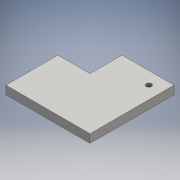
# Autodesk Inventor part: top guide support plate
Saved by Autodesk Inventor 2016 SP1 (Build 200210100, 210)
## iProperties
Created: 2016-05-25
Part Number: top guide support plate
Material: Generic
Document SubType Name: Modeling
Designer: ubik
Density: 1 g/cm^3
Appearance: Default
Author: ubik
Autodesk Inventor part; units mm, degrees
ref_plane "YZ Plane" through (0, 0, 0) normal (1, 0, 0) x (0, 1, 0)
ref_plane "XZ Plane" through (0, 0, 0) normal (0, 1, 0) x (-1, 0, 0)
ref_plane "XY Plane" through (0, 0, 0) normal (0, 0, 1) x (1, 0, 0)
sketch "Sketch1" plane through (0, 0, 0) normal (0, 0, 1) x (1, 0, 0)
  line L0 (-40, 40) -> (40, 40)
  line L1 (40, 40) -> (40, -40)
  line L2 (40, -40) -> (-40, -40)
  line L3 (-40, -40) -> (-40, 40)
  point P0 (0, 0)
  dimension "d0" = 80
  dimension "d1" = 80
  dimension "d4" = 40
  dimension "d5" = 40
  constraints: 8 end point, 2 parallel, 1 horizontal, 1 perpendicular
  measures "d0" distance of L0.start L0.end
  measures "d1" distance of L2.end L0.start
  measures "d4" distance from line of point (0, 0) L3
  measures "d5" distance from line of point (0, 0) L0
extrude "Extrusion1" add sketch "Sketch1" along normal blind 8
sketch "Sketch2" plane through (0, 0, 8) normal (0, 0, 1) x (1, 0, 0)
  circle A0 centre (28, 28) radius 2.5
  line L0 (40, 40) -> (-40, 40) projected
  line L1 (40, -40) -> (40, 40) projected
  point P0 (0, 0)
  dimension "d6" = 5
  dimension "d7" = 12
  dimension "d8" = 12
  constraints: 1 centre point
  measures "d6" diameter of A0
  measures "d7" distance from line of L1 A0.centre
  measures "d8" distance from line of L0 A0.centre
extrude "Extrusion2" cut sketch "Sketch2" against normal through all
sketch "Sketch3" plane through (0, 0, 0) normal (0, 0, -1) x (-1, 0, 0)
  circle A0 centre (-28, 28) radius 2.5 projected
  circle A1 centre (-28, 28) radius 8
  point P0 (0, 0)
  dimension "d11" = 16
  constraints: 1 centre point, 1 coincident
  measures "d11" diameter of A1
extrude "Extrusion3" cut sketch "Sketch3" against normal blind 5
sketch "Sketch4" plane through (0, 0, 0) normal (0, 0, -1) x (-1, 0, 0)
  line L0 (40, 40) -> (-40, 40) projected
  line L1 (9.5, 40) -> (40, 40)
  line L2 (40, 40) -> (40, 9.5)
  line L3 (40, 9.5) -> (9.5, 9.5)
  line L4 (9.5, 9.5) -> (9.5, 40)
  line L5 (40, 40) -> (40, -40) projected
  point P0 (0, 0)
  dimension "d14" = 30.5
  dimension "d15" = 30.5
  dimension "d16" = 0
  constraints: 8 end point, 2 parallel, 1 horizontal, 1 perpendicular, 1 point on line
  measures "d14" distance of L3.end L1.start
  measures "d15" distance of L2.end L3.end
  measures "d16" distance between parallel lines of L5 L2
extrude "Extrusion4" cut sketch "Sketch4" against normal through all
equation "\"d4\" = 0.5 * d0"
equation "\"d5\" = 0.5 * d1"
equation "\"d8\" = d7"
body "Solid1"
